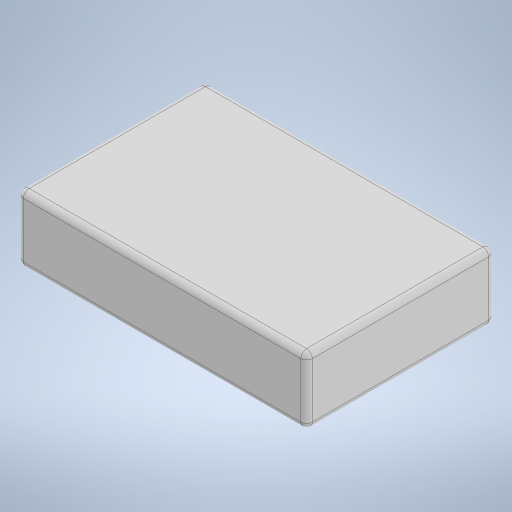
# Autodesk Inventor part: Battery 2023
Saved by Autodesk Inventor 2023 (Build 270158000, 158)
## iProperties
Created: 2024-10-01
Part Number: Battery 2023
Material: Generic
Document SubType Name: Modeling
Designer: bw1293
Density: 1 g/cm^3
Appearance: Default
Author: bw1293
Autodesk Inventor part; units mm, degrees
ref_plane "YZ Plane" through (0, 0, 0) normal (1, 0, 0) x (0, 1, 0)
ref_plane "XZ Plane" through (0, 0, 0) normal (0, 1, 0) x (-1, 0, 0)
ref_plane "XY Plane" through (0, 0, 0) normal (0, 0, 1) x (1, 0, 0)
sketch "Sketch1" plane through (0, 0, 0) normal (0, 1, 0) x (-1, 0, 0)
  line L0 (-50, 32.5) -> (50, 32.5)
  line L1 (50, 32.5) -> (50, -32.5)
  line L2 (50, -32.5) -> (-50, -32.5)
  line L3 (-50, -32.5) -> (-50, 32.5)
  line L4 (-50, 32.5) -> (50, -32.5) construction
  line L5 (50, 32.5) -> (-50, -32.5) construction
  point P0 (0, 0)
  dimension "d0" = 100
  dimension "d1" = 65
  constraints: 12 end point, 2 midpoint, 2 parallel, 1 horizontal, 1 perpendicular
  measures "d0" distance of L1.end L2.end
  measures "d1" distance of L0.end L1.end
extrude "Extrusion1" add sketch "Sketch1" along normal blind 23
fillet "Fillet1" radius 2 12 edges at (0, 23, 32.5) (-50, 23, 0) (0, 23, -32.5) (50, 23, 0) (50, 11.5, 32.5) (50, 11.5, -32.5) (50, 0, 0) (0, 0, 32.5) (-50, 11.5, 32.5) (0, 0, -32.5) (-50, 0, 0) (-50, 11.5, -32.5)
body "Solid1"
